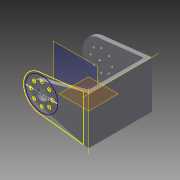
# Autodesk Inventor part: Turnmount
Saved by Autodesk Inventor 2015 (Build 190159000, 159)
## iProperties
Created: 2016-12-14
Part Number: Turnmount
Material: Generic
Document SubType Name: Modeling
Designer: Rudge-Top
Density: 1 g/cm^3
Appearance: Default
Author: Rudge-Top
Autodesk Inventor part; units mm, degrees
ref_plane "YZ Plane" through (0, 0, 0) normal (1, 0, 0) x (0, 1, 0)
ref_plane "XZ Plane" through (0, 0, 0) normal (0, 1, 0) x (-1, 0, 0)
ref_plane "XY Plane" through (0, 0, 0) normal (0, 0, 1) x (1, 0, 0)
sketch "Sketch1" plane through (0, 0, 0) normal (0, 1, 0) x (-1, 0, 0)
  circle A0 centre (0, 0) radius 11.05
  circle A1 centre (0, 0) radius 12.05
  dimension "d0" = 22.1
  dimension "d1" = 24.1
  constraints: 2 centre point, 2 coincident
  measures "d0" diameter of A0
  measures "d1" diameter of A1
extrude "Extrusion1" add sketch "Sketch1" along normal blind 1
sketch "Sketch2" plane through (0, 1, 0) normal (0, 1, 0) x (1, 0, 0)
  arc A0 (0, 13.5) -> (0, -13.5) centre (0, 0) ccw
  line L0 (0, -13.5) -> (32, -13.5)
  line L1 (0, 13.5) -> (32, 13.5) construction
  line L2 (32, -13.5) -> (32, 13.5)
  line L3 (32, -13.5) -> (35, -13.5)
  line L4 (35, -13.5) -> (35, 13.5)
  line L5 (35, 13.5) -> (32, 13.5)
  line L6 (32, 13.5) -> (0, 13.5)
  line L7 (0, -13.5) -> (35, -17.5)
  line L8 (35, -17.5) -> (35, -13.5)
  line L9 (0, 13.5) -> (35, 17.5)
  line L10 (35, 17.5) -> (35, 13.5)
  dimension "d4" = 27
  dimension "d6" = 3
  dimension "d32" = 32
  dimension "d37" = 4
  dimension "d38" = 4
  constraints: 22 end point, 3 horizontal, 3 vertical, 2 perpendicular, 2 point on circle, 1 centre point, 1 coincident, 1 collinear, 1 tangent
  measures "d4" diameter of A0
  measures "d6" distance of L0.end L3.end
  measures "d32" distance of L0.start L0.end
  measures "d37" distance of L7.end L3.end
  measures "d38" distance of L9.end L4.end
extrude "Extrusion2" add sketch "Sketch2" along normal blind 3
sketch "Sketch3" plane through (0, 1, 0) normal (0, -1, 0) x (1, 0, 0)
  circle A0 centre (0, 0) radius 8
  point P0 (-8, 0)
  point P1 (-5.6569, -5.6569)
  point P2 (0, -8)
  point P3 (5.6569, -5.6569)
  point P4 (8, 0)
  point P5 (5.6569, 5.6569)
  point P6 (0, 8)
  point P7 (-5.6569, 5.6569)
  dimension "d9" = 16
  dimension "d12" = 360
  constraints: 1 coincident, 1 horizontal alignment, 11 other
hole "Hole1" at (-8, 1, 0) at (-5.6569, 1, -5.6569) at (0, 1, -8) at (5.6569, 1, -5.6569) at (8, 1, 0) at (5.6569, 1, 5.6569) at (0, 1, 8) at (-5.6569, 1, 5.6569) direction (0, 1, 0) diameter 2.3 end through all
sketch "Sketch4" plane through (0, 0, 0) normal (0, -1, 0) x (1, 0, 0)
  point P0 (0, 0)
sketch "Sketch5" plane through (0, 1, 0) normal (0, -1, 0) x (1, 0, 0)
  arc A0 (0, 13.5) -> (0, -13.5) centre (0, 0) ccw projected
  line L0 (35, 17.5) -> (35, -17.5) projected
  circle A1 centre (0, 0) radius 12.05 projected
  line L1 (35, -13.5) -> (32, -13.5)
  line L2 (32, -13.5) -> (32, 13.5)
  line L3 (32, 13.5) -> (35, 13.5)
  line L4 (35, 13.5) -> (35, -13.5)
  line L5 (0, 13.5) -> (35, 17.5) projected
  line L6 (35, -17.5) -> (0, -13.5) projected
  line L7 (32, -13.5) -> (32, -17.1571)
  line L8 (32, 13.5) -> (32, 17.1571)
  line L9 (32, 17.1571) -> (35, 17.5)
  line L10 (35, 17.5) -> (35, 13.5)
  line L11 (35, 17.5) -> (35, -17.5) projected
  line L12 (35, -13.5) -> (35, -17.5)
  line L13 (35, -17.5) -> (32, -17.1571)
  line L14 (35, -17.5) -> (0, -13.5) projected
  dimension "d21" = 3
  constraints: 20 end point, 4 collinear, 2 parallel, 2 point on line, 2 vertical, 1 horizontal, 1 perpendicular
  measures "d21" distance of L2.end L3.end
extrude "Extrusion3" add sketch "Sketch5" along normal blind 44.1 contours L5 L0 L3 L8 | L7 L1 L0 L6 | L3 L0 L1 L2
ref_plane "Work Plane1" through (0, -19.55, 0) normal (0, 1, 0) x (1, 0, 0)
mirror "Mirror1" about plane through (0, -19.55, 0) normal (0, 1, 0) of "Extrusion2"
sketch "Sketch7" plane through (0, -43.1, 0) normal (0, -1, 0) x (1, 0, 0)
  point P0 (0, 0)
  point P1 (0, 0)
  constraints: 1 coincident
hole "Hole2" at (0, -43.1, 0) direction (0, 1, 0) diameter 8.7 depth 3 tip angle 118
fillet "Fillet1" radius 1 2 edges at (32, 1, 0) (32, -40.1, 0)
sketch "Sketch9" plane through (32, -39.1, 13.5) normal (-1, 0, 0) x (0, 0, 1)
  line L0 (-15.4003, 14.3637) -> (-15.4003, 24.9437) construction
  line L1 (-15.4003, 24.9437) -> (-11.7688, 24.9437) construction
  line L2 (-11.7688, 24.9437) -> (-11.7688, 14.3637) construction
  line L3 (-11.7688, 14.3637) -> (-15.4003, 14.3637) construction
  line L4 (-13.1185, 16.8257) -> (-12.7524, 16.8257)
  line L5 (-12.7524, 16.8257) -> (-12.7524, 16.3567)
  line L6 (-12.7524, 16.3567) -> (-11.8288, 16.3567)
  line L7 (-11.8288, 16.3567) -> (-11.8288, 15.9307)
  line L8 (-11.8288, 15.9307) -> (-12.7524, 15.9307)
  line L9 (-12.7524, 15.9307) -> (-12.7524, 14.4466)
  line L10 (-12.7524, 14.4466) -> (-13.0813, 14.4466)
  line L11 (-13.0813, 14.4466) -> (-15.4003, 16.0736)
  line L12 (-15.4003, 16.0736) -> (-15.4003, 16.3567)
  line L13 (-15.4003, 16.3567) -> (-13.1185, 16.3567)
  line L14 (-13.1185, 16.3567) -> (-13.1185, 16.8257)
  line L15 (-13.1185, 15.9307) -> (-14.857, 15.9307)
  line L16 (-14.857, 15.9307) -> (-13.1185, 14.7011)
  line L17 (-13.1185, 14.7011) -> (-13.1185, 15.9307)
  line L18 (-12.5008, 19.4335) -> (-11.8288, 19.1876)
  line L19 (-11.8288, 19.1876) -> (-11.8288, 17.1231)
  line L20 (-11.8288, 17.1231) -> (-11.9232, 17.1231)
  spline S0 degree 2 poles (-11.9232, 17.1231) (-12.7553, 18.0352) (-13.8076, 18.7787) (-14.2451, 18.7787) knots 0 0 0 1 2 2 2
  spline S1 degree 2 poles (-14.2451, 18.7787) (-14.5768, 18.7787) (-15.0057, 18.3698) (-15.0057, 18.0867) knots 0 0 0 1 2 2 2
  spline S2 degree 2 poles (-15.0057, 18.0867) (-15.0057, 17.8265) (-14.7026, 17.4176) (-14.4109, 17.3175) knots 0 0 0 1 2 2 2
  line L21 (-14.4109, 17.3175) -> (-14.4109, 17.2232)
  spline S3 degree 2 poles (-14.4109, 17.2232) (-14.8885, 17.2889) (-15.4003, 17.8208) (-15.4003, 18.2211) knots 0 0 0 1 2 2 2
  spline S4 degree 2 poles (-15.4003, 18.2211) (-15.4003, 18.6472) (-14.8542, 19.2191) (-14.4824, 19.2191) knots 0 0 0 1 2 2 2
  spline S5 degree 2 poles (-14.4824, 19.2191) (-14.2165, 19.2191) (-13.9506, 19.0961) knots 0 0 0 1 1 1
  spline S6 degree 2 poles (-13.9506, 19.0961) (-13.5331, 18.9045) (-13.0641, 18.4756) knots 0 0 0 1 1 1
  spline S7 degree 2 poles (-13.0641, 18.4756) (-12.3636, 17.8322) (-12.2177, 17.6721) knots 0 0 0 1 1 1
  line L22 (-12.2177, 17.6721) -> (-12.2177, 18.5871)
  spline S8 degree 2 poles (-12.2177, 18.5871) (-12.2177, 18.8674) (-12.2578, 19.0904) (-12.3864, 19.2705) (-12.5008, 19.3392) knots 0 0 0 1 2 3 3 3
  line L23 (-12.5008, 19.3392) -> (-12.5008, 19.4335)
  spline S9 degree 2 poles (-13.5588, 19.8453) (-14.1564, 19.8453) (-15.02, 20.2056) (-15.2316, 20.5058) knots 0 0 0 1 2 2 2
  spline S10 degree 2 poles (-15.2316, 20.5058) (-15.4003, 20.7375) (-15.4003, 20.9862) knots 0 0 0 1 1 1
  spline S11 degree 2 poles (-15.4003, 20.9862) (-15.4003, 21.3894) (-14.9914, 21.7097) knots 0 0 0 1 1 1
  spline S12 degree 2 poles (-14.9914, 21.7097) (-14.4824, 22.11) (-13.6131, 22.11) knots 0 0 0 1 1 1
  spline S13 degree 2 poles (-13.6131, 22.11) (-13.0041, 22.11) (-12.152, 21.7583) (-11.7688, 21.215) (-11.7688, 20.9605) knots 0 0 0 1 2 3 3 3
  spline S14 degree 2 poles (-11.7688, 20.9605) (-11.7688, 20.4601) (-12.3607, 20.1255) knots 0 0 0 1 1 1
  spline S15 degree 2 poles (-12.3607, 20.1255) (-12.8582, 19.8453) (-13.5588, 19.8453) knots 0 0 0 1 1 1
  spline S16 degree 2 poles (-13.4931, 20.3514) (-12.7725, 20.3514) (-12.3149, 20.5287) knots 0 0 0 1 1 1
  spline S17 degree 2 poles (-12.3149, 20.5287) (-11.9318, 20.6774) (-11.9318, 20.9691) knots 0 0 0 1 1 1
  spline S18 degree 2 poles (-11.9318, 20.9691) (-11.9318, 21.1092) (-12.1806, 21.4066) (-12.4751, 21.4838) knots 0 0 0 1 2 2 2
  spline S19 degree 2 poles (-12.4751, 21.4838) (-12.9183, 21.6039) (-13.7247, 21.6039) knots 0 0 0 1 1 1
  spline S20 degree 2 poles (-13.7247, 21.6039) (-14.3252, 21.6039) (-14.7226, 21.4809) knots 0 0 0 1 1 1
  spline S21 degree 2 poles (-14.7226, 21.4809) (-15.02, 21.3866) (-15.143, 21.2407) knots 0 0 0 1 1 1
  spline S22 degree 2 poles (-15.143, 21.2407) (-15.2288, 21.1349) (-15.2288, 20.9834) knots 0 0 0 1 1 1
  spline S23 degree 2 poles (-15.2288, 20.9834) (-15.2288, 20.8089) (-15.0715, 20.6717) knots 0 0 0 1 1 1
  spline S24 degree 2 poles (-15.0715, 20.6717) (-14.857, 20.4858) (-13.9391, 20.3514) (-13.4931, 20.3514) knots 0 0 0 1 2 2 2
  line L24 (-12.5008, 24.7236) -> (-11.8288, 24.4776)
  line L25 (-11.8288, 24.4776) -> (-11.8288, 22.4131)
  line L26 (-11.8288, 22.4131) -> (-11.9232, 22.4131)
  spline S25 degree 2 poles (-11.9232, 22.4131) (-12.7553, 23.3253) (-13.8076, 24.0687) (-14.2451, 24.0687) knots 0 0 0 1 2 2 2
  spline S26 degree 2 poles (-14.2451, 24.0687) (-14.5768, 24.0687) (-15.0057, 23.6598) (-15.0057, 23.3768) knots 0 0 0 1 2 2 2
  spline S27 degree 2 poles (-15.0057, 23.3768) (-15.0057, 23.1165) (-14.7026, 22.7076) (-14.4109, 22.6076) knots 0 0 0 1 2 2 2
  line L27 (-14.4109, 22.6076) -> (-14.4109, 22.5132)
  spline S28 degree 2 poles (-14.4109, 22.5132) (-14.8885, 22.579) (-15.4003, 23.1108) (-15.4003, 23.5111) knots 0 0 0 1 2 2 2
  spline S29 degree 2 poles (-15.4003, 23.5111) (-15.4003, 23.9372) (-14.8542, 24.5091) (-14.4824, 24.5091) knots 0 0 0 1 2 2 2
  spline S30 degree 2 poles (-14.4824, 24.5091) (-14.2165, 24.5091) (-13.9506, 24.3861) knots 0 0 0 1 1 1
  spline S31 degree 2 poles (-13.9506, 24.3861) (-13.5331, 24.1946) (-13.0641, 23.7656) knots 0 0 0 1 1 1
  spline S32 degree 2 poles (-13.0641, 23.7656) (-12.3636, 23.1223) (-12.2177, 22.9621) knots 0 0 0 1 1 1
  line L28 (-12.2177, 22.9621) -> (-12.2177, 23.8772)
  spline S33 degree 2 poles (-12.2177, 23.8772) (-12.2177, 24.1574) (-12.2578, 24.3804) (-12.3864, 24.5606) (-12.5008, 24.6292) knots 0 0 0 1 2 3 3 3
  line L29 (-12.5008, 24.6292) -> (-12.5008, 24.7236)
  point P0 (-13.5, 39.1)
  constraints: 2 other
extrude "Extrusion4" add sketch "Sketch9" along normal blind 0.5
sketch "Sketch10" plane through (0, -43.1, 0) normal (0, -1, 0) x (1, 0, 0)
  circle A0 centre (0, 0) radius 4.35 projected
  line L0 (35, -17.5) -> (35, 17.5) projected
  arc A1 (0, 13.5) -> (0, -13.5) centre (0, 0) ccw projected
  circle A2 centre (-8, 0) radius 1.15 projected
  arc A3 (0, 13.5) -> (0, -13.5) centre (7.3906, 0) ccw
  line L1 (35, 17.5) -> (0, 13.5) projected
  line L2 (35, -17.5) -> (0, -13.5) projected
  constraints: 3 point on circle, 1 centre point
extrude "Extrusion5" cut sketch "Sketch10" against normal blind 10 contours A1 A3 A2 | A2 A3 picked at (-8.3772, -0.0473)
ref_plane "Work Plane2" through (35, -43.1, 17.5) normal (0, 0, 1) x (1, 0, 0)
sketch "Sketch11" plane through (0, 0, 0) normal (0, -1, 0) x (1, 0, 0)
  line L0 (18.1955, -23.431) -> (-32.443, -23.431)
  line L1 (-32.443, -23.431) -> (-32.443, 30.1256)
  line L2 (-32.443, 30.1256) -> (18.1955, 30.1256)
  line L3 (18.1955, 30.1256) -> (18.1955, -23.431)
  point P0 (0, 0)
  constraints: 8 end point, 2 parallel, 1 horizontal, 1 perpendicular
extrude "Extrusion6" cut sketch "Sketch11" against normal blind 1
sketch "Sketch12" plane through (0, -43.1, 0) normal (0, -1, 0) x (1, 0, 0)
  circle A0 centre (-8, 0) radius 1.15 projected
  arc A1 (-2.1689, 7.7004) -> (-2.1689, -7.7004) centre (0, 0) ccw
  line L0 (-8, 0) -> (0, 0)
  arc A2 (0, 13.5) -> (0, -13.5) centre (7.3906, 0) ccw projected
  line L1 (35, -17.5) -> (0, -13.5) projected
  line L2 (35, -17.5) -> (35, 17.5) projected
  line L3 (35, 17.5) -> (0, 13.5) projected
  circle A3 centre (0, 0) radius 4.35 projected
  line L4 (35, -17.5) -> (35, 17.5)
  line L5 (35, 17.5) -> (35, -17.5) projected
  line L6 (31, 17.0429) -> (31, -17.0429) projected
  line L7 (31, -17.0429) -> (-2.1689, -7.7004)
  line L8 (31, 17.0429) -> (-2.1689, 7.7004)
  line L9 (31, -17.0429) -> (31, 17.0429)
  point P0 (35, 17.5)
  constraints: 10 end point, 3 point on circle, 2 collinear, 2 symmetric about line, 1 centre point, 1 coincident, 1 horizontal, 1 tangent
extrude "Extrusion7" cut sketch "Sketch12" against normal blind 10 contours A1 A2 A0 | A0 A2 L3 L8 A1 | A1 L7 L1 A2 A0 | A0 A2 A1
sketch "Sketch13" plane through (0, -43.1, 0) normal (0, -1, 0) x (1, 0, 0)
  line L0 (31, -17.0429) -> (0, -13.5) projected
  line L1 (31, 17.0429) -> (31, -17.0429) projected
  line L2 (0, 13.5) -> (31, 17.0429) projected
  arc A0 (0, 13.5) -> (0, -13.5) centre (0, 0) ccw projected
  circle A1 centre (0, 8) radius 1.15 projected
  circle A2 centre (8, 0) radius 1.15 projected
  circle A3 centre (0, -8) radius 1.15 projected
  circle A4 centre (-8, 0) radius 1.15 projected
  circle A5 centre (-5.6569, -5.6569) radius 1.15 projected
  circle A6 centre (5.6569, -5.6569) radius 1.15 projected
  circle A7 centre (5.6569, 5.6569) radius 1.15 projected
  circle A8 centre (-5.6569, 5.6569) radius 1.15 projected
  circle A9 centre (0, 0) radius 12
  dimension "d43" = 24
  constraints: 1 centre point, 1 coincident
  measures "d43" diameter of A9
body "Solid1"
